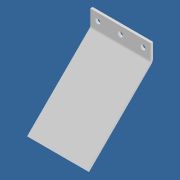
# Autodesk Inventor part: Fan_Holder
Saved by Autodesk Inventor 2020 (Build 240168000, 168)
## iProperties
Created: 2021-06-06
Part Number: Fan_Holder
Material: 一般
Document SubType Name: Sheet Metal
Designer: ken113
Density: 1 g/cm^3
Sheet Metal Rule: Default_mm
Appearance: 既定
Author: ken113
Autodesk Inventor part; units mm, degrees
ref_plane "YZ Plane" through (0, 0, 0) normal (1, 0, 0) x (0, 1, 0)
ref_plane "XZ Plane" through (0, 0, 0) normal (0, 1, 0) x (-1, 0, 0)
ref_plane "XY Plane" through (0, 0, 0) normal (0, 0, 1) x (1, 0, 0)
sketch "スケッチ1" plane through (0, 0, 0) normal (0, 0, 1) x (1, 0, 0)
  line L0 (20, 0) -> (-20, 0)
  line L1 (-20, 0) -> (-20, 10)
  line L2 (-20, 10) -> (20, 10)
  line L3 (20, 10) -> (20, 0)
  line L4 (20, 0) -> (-20, 10) construction
  line L5 (-20, 0) -> (20, 10) construction
  point P0 (0, 0)
  point P1 (0, 5)
  point P2 (0, 0)
  point P3 (0, 5)
  dimension "d0" = 40
  dimension "d1" = 10
  measures "d0" distance of L1.end L2.end
  measures "d1" distance of L0.end L1.end
extrude "プレート1" add sketch "スケッチ1" along normal blind 1.6
sketch "スケッチ2" plane through (20, -1.1314, 2.0686) normal (0, -0.7071068, -0.7071068) x (1, 0, 0)
  line L0 (-40, 0) -> (0, 0)
  line L1 (0, 0) -> (0, 58.6745)
  line L2 (0, 58.6745) -> (-40, 58.6745)
  line L3 (-40, 58.6745) -> (-40, 0)
  constraints: 6 end point, 1 horizontal, 1 perpendicular, 1 vertical
edge flange "フランジ1" height 60 angle 45 thickness 1.6 bend radius 1.6 thickness toward (0, -0.7071068, -0.7071068) relief straight relief width 1.6 relief depth 0.8 edges at (0, 0, 1.6) wall of the first edge with corners at (-20, -1.1314, 2.0686) (20, -1.1314, 2.0686) (20, -42.6205, 43.5578) (-20, -42.6205, 43.5578)
bend "曲げ1"
corner "コーナー1"
sketch "スケッチ3" plane through (0, 0, 0) normal (0, 0, -1) x (-1, 0, 0)
  line L0 (-20, 0) -> (20, 0) projected
  line L1 (20, 0) -> (20, 10) projected
  line L2 (20, 10) -> (-20, 10) projected
  line L3 (-20, 10) -> (-20, 0) projected
  point P0 (0, 0)
  point P1 (-15, 5)
  point P2 (15, 5)
  point P3 (0, 5)
  point P4 (0, 0)
  dimension "d13" = 5
  dimension "d14" = 5
  dimension "d15" = 5
  constraints: 2 horizontal alignment, 1 midpoint, 1 vertical alignment
  measures "d13" distance from line of L2 point (-15, 5)
  measures "d14" distance from line of point (-15, 5) L3
  measures "d15" distance from line of L1 point (15, 5)
hole "穴1" at (15, 5, 0) at (-15, 5, 0) at (0, 5, 0) direction (0, 0, 1) diameter 3.2 depth 1.6 tip angle 118
equation "\"d21\" = Thickness"
equation "\"d2\" = Thickness"
equation "\"d3\" = BendReliefWidth"
equation "\"d4\" = BendReliefDepth"
equation "\"d5\" = MinimumRemnant"
equation "\"d6\" = TransitionRadius"
equation "\"d9\" = BendRadius"
equation "\"d10\" = CornerReliefSize"
equation "\"d11\" = GapSize"
equation "\"d12\" = JacobiRadiusSize"
equation "\"BendRadius\" = Thickness"
equation "\"BendReliefWidth\" = Thickness"
equation "\"BendReliefDepth\" = 0.5 * Thickness"
equation "\"CornerReliefSize\" = 4 * Thickness"
equation "\"MinimumRemnant\" = 2 * Thickness"
equation "\"TransitionRadius\" = BendRadius"
equation "\"JacobiRadiusSize\" = BendRadius"
equation "\"GapSize\" = Thickness"
equation "\"Thickness\" = 1.6"
